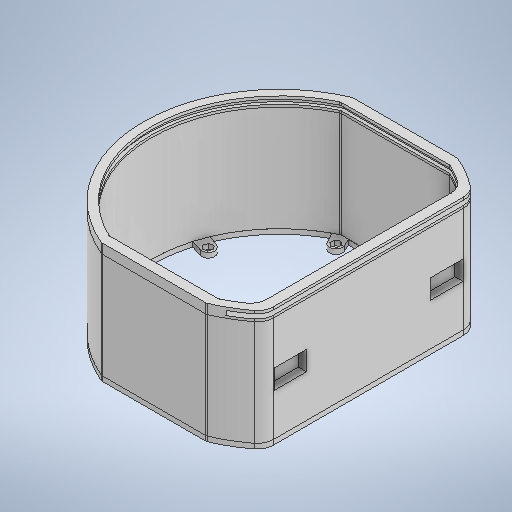
# Autodesk Inventor part: carcasa4.0
Saved by Autodesk Inventor 2025.3 (Build 293356030, 356C)
## iProperties
Created: 2025-08-27
Part Number: carcasa4.0
Material: Generic
Document SubType Name: Modeling
Designer: cdavi
Density: 1 g/cm^3
Appearance: Default
Author: cdavi
Autodesk Inventor part; units mm, degrees
ref_plane "YZ Plane" through (0, 0, 0) normal (1, 0, 0) x (0, 1, 0)
ref_plane "XZ Plane" through (0, 0, 0) normal (0, 1, 0) x (-1, 0, 0)
ref_plane "XY Plane" through (0, 0, 0) normal (0, 0, 1) x (1, 0, 0)
sketch "Sketch1" plane through (0, 0, 0) normal (0, 1, 0) x (-1, 0, 0)
  line L0 (33.1474, 71.5) -> (-33.1474, 71.5)
  line L1 (0, 0) -> (-55, 0) construction
  line L2 (31.9961, 77.5) -> (-31.9961, 77.5)
  line L3 (33.1474, -71.5) -> (-33.5969, -71.5)
  line L4 (31.9961, -77.5) -> (-31.9961, -77.5)
  line L5 (0, 0) -> (0, 77.5) construction
  line L6 (-49, 56.921) -> (-49, -56.921)
  line L7 (-55, 58.7452) -> (-55, -58.7452)
  arc A0 (-44.6522, -65.1704) -> (-33.5969, -71.5) centre (0, 0) ccw
  arc A1 (-51.0811, -66.6838) -> (-32.7765, -77.3415) centre (0, 0) ccw
  arc A2 (32.7765, -77.3415) -> (32.7765, 77.3415) centre (0, 0) ccw
  arc A3 (-32.7765, 77.3415) -> (-51.0811, 66.6838) centre (0, 0) ccw
  arc A4 (34.0084, -71.3052) -> (34.0084, 71.3052) centre (0, 0) ccw
  arc A5 (-34.0084, 71.3052) -> (-44.6522, 65.1704) centre (0, 0) ccw
  arc A6 (-32.7765, -77.3415) -> (-31.9961, -77.5) centre (-31.9961, -75.5) ccw
  arc A7 (31.9961, -77.5) -> (32.7765, -77.3415) centre (31.9961, -75.5) ccw
  arc A8 (33.1474, -71.5) -> (34.0084, -71.3052) centre (33.1474, -69.5) ccw
  arc A9 (34.0084, 71.3052) -> (33.1474, 71.5) centre (33.1474, 69.5) ccw
  arc A10 (32.7765, 77.3415) -> (31.9961, 77.5) centre (31.9961, 75.5) ccw
  arc A11 (-33.1474, 71.5) -> (-34.0084, 71.3052) centre (-33.1474, 69.5) ccw
  arc A12 (-31.9961, 77.5) -> (-32.7765, 77.3415) centre (-31.9961, 75.5) ccw
  arc A13 (-44.6522, 65.1704) -> (-49, 56.921) centre (-39, 56.921) ccw
  arc A14 (-51.0811, 66.6838) -> (-55, 58.7452) centre (-45, 58.7452) ccw
  arc A15 (-55, -58.7452) -> (-51.0811, -66.6838) centre (-45, -58.7452) ccw
  arc A16 (-49, -56.921) -> (-44.6522, -65.1704) centre (-39, -56.921) ccw
  point P0 (-32.3998, 77.5)
  point P1 (33.5969, -71.5)
  point P2 (32.3998, -77.5)
  point P3 (-32.3998, -77.5)
  point P4 (-55, -63.4902)
  point P5 (-49, 61.9677)
  point P6 (-49, -61.9677)
  point P7 (-55, 63.4902)
  point P8 (32.3998, 77.5)
  point P9 (33.5969, 71.5)
  point P10 (-33.5969, 71.5)
  dimension "d2" = 71.5
  dimension "d4" = 6
  dimension "d6" = 49
  dimension "d7" = 6
  dimension "d8" = 2
  dimension "d9" = 10
  dimension "d10" = 79
  dimension "d11" = 84
  dimension "d12" = 79
  dimension "d13" = 84
  constraints: 45 point on circle, 22 tangent, 17 centre point, 16 end point, 11 point on line, 9 equal radius, 4 symmetric about line, 3 vertical, 2 coincident, 2 horizontal, 2 midpoint, 1 parallel
  measures "d2" distance between parallel lines of L1 L0
  measures "d4" distance between parallel lines of L0 L2
  measures "d6" distance between parallel lines of L6 L5
  measures "d7" distance between parallel lines of L7 L6
  measures "d8" radius of A6
  measures "d9" radius of A13
  measures "d10" radius of A4
  measures "d11" radius of A2
  measures "d12" radius of A0
  measures "d13" radius of A1
extrude "Extrusion1" add sketch "Sketch1" along normal blind 65
sketch "Sketch2" plane through (55, 0, 58.7452) normal (1, 0, 0) x (0, 0, -1)
  line L0 (58.7452, 0) -> (58.7452, 65) construction
  line L1 (115.6662, 65) -> (1.8242, 65) projected
  line L2 (0.4037, 38) -> (20.4037, 38)
  line L3 (20.4037, 38) -> (20.4037, 26)
  line L4 (20.4037, 26) -> (0.4037, 26)
  line L5 (0.4037, 26) -> (0.4037, 38)
  line L6 (0, 0) -> (117.4904, 0) projected
  line L7 (-18.5963, 0) -> (-18.5963, 65) projected
  line L8 (117.0867, 38) -> (97.0867, 38)
  line L9 (97.0867, 38) -> (97.0867, 26)
  line L10 (97.0867, 26) -> (117.0867, 26)
  line L11 (117.0867, 26) -> (117.0867, 38)
  dimension "d16" = 26
  dimension "d17" = 19
  dimension "d18" = 12
  dimension "d19" = 20
  constraints: 18 end point, 4 symmetric about line, 2 parallel, 1 horizontal, 1 midpoint, 1 perpendicular
  measures "d16" distance between parallel lines of L6 L4
  measures "d17" distance between parallel lines of L5 L7
  measures "d18" distance of L2.end L3.end
  measures "d19" distance of L2.start L2.end
extrude "Extrusion2" cut sketch "Sketch2" against normal blind 5
sketch "Sketch3" plane through (55, 0, 58.7452) normal (1, 0, 0) x (0, 0, -1)
  line L0 (3.568, 49.2223) -> (17.7975, 43.9952) construction
  line L1 (2.8909, 47.379) -> (17.1204, 42.1519)
  line L2 (18.4746, 45.8385) -> (4.2452, 51.0656)
  arc A0 (4.2452, 51.0656) -> (2.8909, 47.379) centre (3.568, 49.2223) ccw
  arc A1 (17.1204, 42.1519) -> (18.4746, 45.8385) centre (17.7975, 43.9952) ccw
  arc A2 (44.4296, 11.624) -> (34.6921, 2.9774) centre (43.8866, 2.4292) ccw construction
  arc A3 (44.531, 13.3402) -> (32.9759, 3.0797) centre (43.8866, 2.4292) ccw
  arc A4 (44.3283, 9.9077) -> (36.4083, 2.8751) centre (43.8866, 2.4292) ccw
  arc A5 (44.3283, 9.9077) -> (44.531, 13.3402) centre (44.4296, 11.624) ccw
  arc A6 (32.9759, 3.0797) -> (36.4083, 2.8751) centre (34.6921, 2.9774) ccw
  line L3 (58.7452, 0) -> (58.7452, 65) construction
  line L4 (114.5995, 47.379) -> (100.3701, 42.1519)
  line L5 (99.0158, 45.8385) -> (113.2453, 51.0656)
  arc A7 (114.5995, 47.379) -> (113.2453, 51.0656) centre (113.9224, 49.2223) ccw
  arc A8 (99.0158, 45.8385) -> (100.3701, 42.1519) centre (99.6929, 43.9952) ccw
  point P0 (10.6828, 46.6088)
  constraints: 18 point on circle, 12 end point, 9 centre point, 8 tangent, 6 symmetric about line, 1 midpoint, 1 parallel, 2 other
extrude "Extrusion3" [suppressed]
extrude "Extrusion4" add sketch "Sketch1" along normal blind 3 from surface at 65 separate body contours A9 A4 A8 L3 A0 A16 L6 A13 A5 A11 L0 | A10 A2 A7 L4 A6 A1 A15 L7 A14 A3 A12 L2
sketch "Sketch5" plane through (-31.9961, 68, 77.5) normal (0, 1, 0) x (1, 0, 0)
  circle A0 centre (31.9961, 77.5) radius 8.5
  circle A1 centre (1.9961, 77.5) radius 2.5
  line L0 (40.1201, 75) -> (48.9961, 75)
  line L1 (48.9961, 75) -> (48.9961, 80)
  line L2 (48.9961, 80) -> (40.1201, 80)
  line L3 (48.9961, 77.5) -> (86.9961, 77.5)
  line L4 (86.9961, 18.7548) -> (86.9961, 136.2452) projected
  line L5 (1.9961, 77.5) -> (-52.0039, 77.5)
  arc A2 (-0.7804, 154.8415) -> (-0.7804, 0.1585) centre (31.9961, 77.5) ccw projected
  dimension "d26" = 17
  dimension "d27" = 5
  dimension "d31" = 5
  dimension "d32" = 17
  dimension "d47" = 30
  dimension "d204" = 38
  dimension "d205" = 54
  dimension "d206" = 55
  constraints: 10 end point, 3 point on circle, 2 centre point, 2 horizontal alignment, 2 midpoint, 2 perpendicular, 1 coincident, 1 horizontal, 1 point on line
  measures "d26" diameter of A0
  measures "d27" diameter of A1
  measures "d31" distance between parallel lines of L2 L0
  measures "d32" distance from line of A0.centre L1
  measures "d47" distance of A0.centre L5.start
  measures "d204" distance of L3.start L3.end
  measures "d205" distance of L5.start L5.end
  measures "d206" distance from line of L4 point (31.996, 77.5)
extrude "Extrusion5" cut sketch "Sketch5" against normal through all bodies 2
sketch "Sketch6" plane through (0, 0, 0) normal (0, 1, 0) x (-1, 0, 0)
  circle A0 centre (0, 0) radius 72 construction
  arc A1 (-34.0084, 71.3052) -> (-44.6522, 65.1704) centre (0, 0) ccw projected
  arc A2 (-44.6522, 65.1704) -> (-49, 56.921) centre (-39, 56.921) ccw projected
  line L0 (-49, -56.921) -> (-49, 56.921) projected
  arc A3 (-49, -56.921) -> (-44.6522, -65.1704) centre (-39, -56.921) ccw projected
  arc A4 (-44.6522, -65.1704) -> (-33.5969, -71.5) centre (0, 0) ccw projected
  line L1 (33.1474, -71.5) -> (-33.5969, -71.5) construction
  arc A5 (34.0084, -71.3052) -> (34.0084, 71.3052) centre (0, 0) ccw projected
  line L2 (-33.1474, 71.5) -> (33.1474, 71.5) construction
  line L3 (31.9961, 77.5) -> (-31.9961, 77.5) projected
  arc A6 (-32.7765, 77.3415) -> (-51.0811, 66.6838) centre (0, 0) ccw projected
  arc A7 (-51.0811, 66.6838) -> (-55, 58.7452) centre (-45, 58.7452) ccw projected
  line L4 (-55, 58.7452) -> (-55, -58.7452) projected
  arc A8 (-55, -58.7452) -> (-51.0811, -66.6838) centre (-45, -58.7452) ccw projected
  arc A9 (-51.0811, -66.6838) -> (-32.7765, -77.3415) centre (0, 0) ccw projected
  line L5 (-31.9961, -77.5) -> (31.9961, -77.5) projected
  arc A10 (32.7765, -77.3415) -> (32.7765, 77.3415) centre (0, 0) ccw projected
  arc A11 (-32.6555, 65.2887) -> (-41.2609, 60.2208) centre (0, 0) ccw construction
  arc A12 (-41.2609, 60.2208) -> (-43, 56.921) centre (-39, 56.921) ccw construction
  line L6 (-43, 56.921) -> (-43, -56.921) construction
  arc A13 (-43, -56.921) -> (-41.2609, -60.2208) centre (-39, -56.921) ccw construction
  arc A14 (-41.2609, -60.2208) -> (-32.6555, -65.2887) centre (0, 0) ccw construction
  line L7 (-31.7608, -65.5) -> (31.7608, -65.5) construction
  line L8 (-31.7608, 65.5) -> (31.7608, 65.5) construction
  arc A15 (32.6555, -65.2887) -> (32.6555, 65.2887) centre (0, 0) ccw construction
  arc A16 (-8.124, -2.5) -> (-8.124, 2.5) centre (0, 0) ccw projected
  line L9 (0, 0) -> (67.9077, 23.9278) construction
  line L10 (0, 0) -> (84, 0) construction
  circle A17 centre (67.9077, 23.9278) radius 2.85 construction
  line L11 (0, 0) -> (0, -72) construction
  circle A18 centre (30.4285, 65.2542) radius 2.85 construction
  line L12 (30.4285, 65.2542) -> (0, 0) construction
  circle A19 centre (-45.5, 20) radius 2.85 construction
  circle A20 centre (-30.4285, 65.2542) radius 2.85 construction
  line L13 (-30.4285, 65.2542) -> (0, 0) construction
  arc A21 (-31.7608, 65.5) -> (-32.6555, 65.2887) centre (-31.7608, 63.5) ccw construction
  arc A22 (-32.6555, -65.2887) -> (-31.7608, -65.5) centre (-31.7608, -63.5) ccw construction
  arc A23 (31.7608, -65.5) -> (32.6555, -65.2887) centre (31.7608, -63.5) ccw construction
  arc A24 (32.6555, 65.2887) -> (31.7608, 65.5) centre (31.7608, 63.5) ccw construction
  arc A25 (-32.7765, -77.3415) -> (-31.9961, -77.5) centre (-31.9961, -75.5) ccw projected
  arc A26 (31.9961, -77.5) -> (32.7765, -77.3415) centre (31.9961, -75.5) ccw projected
  arc A27 (32.7765, 77.3415) -> (31.9961, 77.5) centre (31.9961, 75.5) ccw projected
  arc A28 (-31.9961, 77.5) -> (-32.7765, 77.3415) centre (-31.9961, 75.5) ccw projected
  circle A29 centre (67.9077, -23.9278) radius 2.85 construction
  circle A30 centre (30.4285, -65.2542) radius 2.85 construction
  circle A31 centre (-45.5, -20) radius 2.85 construction
  circle A32 centre (-30.4285, -65.2542) radius 2.85 construction
  line L14 (34.0084, 64.5944) -> (34.0084, 71.3052)
  line L15 (-34.0084, 64.5944) -> (-34.0084, 71.3052)
  line L16 (34.0084, 71.3052) -> (-34.0084, 71.3052)
  line L17 (34.0084, -64.5944) -> (34.0084, -71.3052)
  line L18 (-34.0084, -64.5944) -> (-34.0084, -71.3052)
  line L19 (34.0084, -71.3052) -> (-34.0084, -71.3052)
  circle A33 centre (67.9077, 23.9278) radius 4
  circle A34 centre (30.4285, 65.2542) radius 4
  line L20 (65.1063, 24.4516) -> (66.9606, 26.6158)
  line L21 (66.9606, 26.6158) -> (69.762, 26.0921)
  line L22 (69.762, 26.0921) -> (70.7092, 23.4041)
  line L23 (70.7092, 23.4041) -> (68.8549, 21.2398)
  line L24 (68.8549, 21.2398) -> (66.0534, 21.7636)
  line L25 (66.0534, 21.7636) -> (65.1063, 24.4516)
  line L26 (28.0939, 63.6195) -> (27.8455, 66.4586)
  line L27 (27.8455, 66.4586) -> (30.1801, 68.0933)
  line L28 (30.1801, 68.0933) -> (32.7631, 66.8889)
  line L29 (32.7631, 66.8889) -> (33.0115, 64.0497)
  line L30 (33.0115, 64.0497) -> (30.6769, 62.415)
  line L31 (30.6769, 62.415) -> (28.0939, 63.6195)
  circle A35 centre (-45.5, 20) radius 4
  line L32 (-47.9682, 18.575) -> (-47.9682, 21.425)
  line L33 (-47.9682, 21.425) -> (-45.5, 22.85)
  line L34 (-45.5, 22.85) -> (-43.0318, 21.425)
  line L35 (-43.0318, 21.425) -> (-43.0318, 18.575)
  line L36 (-43.0318, 18.575) -> (-45.5, 17.15)
  line L37 (-45.5, 17.15) -> (-47.9682, 18.575)
  line L38 (-45.5, 24) -> (-49, 24)
  line L39 (-45.5, 16) -> (-49, 16)
  circle A36 centre (-30.4285, 65.2542) radius 4
  line L40 (-30.6769, 62.415) -> (-33.0115, 64.0497)
  line L41 (-33.0115, 64.0497) -> (-32.7631, 66.8889)
  line L42 (-32.7631, 66.8889) -> (-30.1801, 68.0933)
  line L43 (-30.1801, 68.0933) -> (-27.8455, 66.4586)
  line L44 (-27.8455, 66.4586) -> (-28.0939, 63.6195)
  line L45 (-28.0939, 63.6195) -> (-30.6769, 62.415)
  line L46 (-34.0054, 63.4636) -> (-37.1399, 69.7254)
  circle A37 centre (67.9077, -23.9278) radius 4
  circle A38 centre (30.4285, -65.2542) radius 4
  circle A39 centre (-45.5, -20) radius 4
  line L47 (-45.5, -24) -> (-49, -24)
  line L48 (-45.5, -16) -> (-49, -16)
  circle A40 centre (-30.4285, -65.2542) radius 4
  line L49 (-34.0054, -63.4636) -> (-37.1399, -69.7254)
  line L50 (65.1063, -24.4516) -> (66.9606, -26.6158)
  line L51 (66.9606, -26.6158) -> (69.762, -26.0921)
  line L52 (69.762, -26.0921) -> (70.7092, -23.4041)
  line L53 (70.7092, -23.4041) -> (68.8549, -21.2398)
  line L54 (68.8549, -21.2398) -> (66.0534, -21.7636)
  line L55 (66.0534, -21.7636) -> (65.1063, -24.4516)
  line L56 (28.0939, -63.6195) -> (27.8455, -66.4586)
  line L57 (27.8455, -66.4586) -> (30.1801, -68.0933)
  line L58 (30.1801, -68.0933) -> (32.7631, -66.8889)
  line L59 (32.7631, -66.8889) -> (33.0115, -64.0497)
  line L60 (33.0115, -64.0497) -> (30.6769, -62.415)
  line L61 (30.6769, -62.415) -> (28.0939, -63.6195)
  line L62 (-30.6769, -62.415) -> (-33.0115, -64.0497)
  line L63 (-33.0115, -64.0497) -> (-32.7631, -66.8889)
  line L64 (-32.7631, -66.8889) -> (-30.1801, -68.0933)
  line L65 (-30.1801, -68.0933) -> (-27.8455, -66.4586)
  line L66 (-27.8455, -66.4586) -> (-28.0939, -63.6195)
  line L67 (-28.0939, -63.6195) -> (-30.6769, -62.415)
  line L68 (-47.9682, -18.575) -> (-47.9682, -21.425)
  line L69 (-47.9682, -21.425) -> (-45.5, -22.85)
  line L70 (-45.5, -22.85) -> (-43.0318, -21.425)
  line L71 (-43.0318, -21.425) -> (-43.0318, -18.575)
  line L72 (-43.0318, -18.575) -> (-45.5, -17.15)
  line L73 (-45.5, -17.15) -> (-47.9682, -18.575)
  line L74 (66.4741, 27.6621) -> (73.0114, 30.1718)
  line L75 (69.1317, 20.1197) -> (75.7983, 22.2625)
  line L76 (34.0054, 63.4636) -> (37.1399, 69.7254)
  line L77 (66.4741, -27.6621) -> (73.0114, -30.1718)
  line L78 (69.1317, -20.1197) -> (75.7983, -22.2625)
  line L79 (34.0054, -63.4636) -> (37.1399, -69.7254)
  line L80 (-26.7577, 66.8433) -> (-29.5397, 73.2694)
  line L81 (26.7577, 66.8433) -> (29.5397, 73.2694)
  line L82 (-26.7577, -66.8433) -> (-29.5397, -73.2694)
  line L83 (26.7577, -66.8433) -> (29.5397, -73.2694)
  line L84 (-33.1474, 71.5) -> (-55, 71.5)
  line L85 (-55, 71.5) -> (-55, 58.7452)
  line L86 (-44.088, 71.5) -> (-33.1474, 71.5)
  point P0 (-32.2296, -65.5)
  point P1 (-34.0084, 64.5944)
  point P2 (30.4285, 65.2542)
  point P3 (-37.1399, -69.7254)
  point P4 (-49, -24)
  point P5 (-49, -16)
  point P6 (75.7983, -22.2625)
  point P7 (69.1317, -20.1197)
  point P8 (66.4741, -27.6621)
  point P9 (73.0114, -30.1718)
  point P10 (34.0054, -63.4636)
  point P11 (-27.1107, 64.5369)
  point P12 (-27.1107, -64.5369)
  point P13 (27.1107, -64.5369)
  point P14 (27.1107, 64.5369)
  point P15 (-49, 21.9365)
  point P16 (-49, 18.0635)
  point P17 (-32.0117, 62.2515)
  point P18 (32.0117, -62.2515)
  point P19 (66.8707, -20.6956)
  point P20 (65.0736, -25.796)
  point P21 (-32.0117, -62.2515)
  point P22 (-49, -21.9365)
  point P23 (-49, -18.0635)
  point P24 (65.0736, 25.796)
  point P25 (66.8707, 20.6956)
  point P26 (32.0117, 62.2515)
  point P27 (25.828, -65.0609)
  point P28 (-25.828, -65.0609)
  point P29 (-26.7577, -66.8433)
  point P30 (34.0084, -67.0387)
  point P31 (-28.6893, -71.3052)
  point P32 (28.6893, -71.3052)
  point P33 (28.6893, 71.3052)
  point P34 (-28.6893, 71.3052)
  point P35 (34.0084, 67.0387)
  point P36 (-34.0084, -71.3052)
  point P37 (-34.0084, -67.0387)
  point P38 (-34.0084, 67.0387)
  dimension "d33" = 144
  dimension "d39" = 5.7
  dimension "d34" = 6
  dimension "d35" = 6
  dimension "d36" = 6
  dimension "d37" = 19.41
  dimension "d38" = 25
  dimension "d40" = 20
  dimension "d41" = 3.5
  dimension "d42" = 25
  dimension "d44" = 2
  dimension "d61" = 8
  dimension "d62" = 8
  dimension "d63" = 8
  dimension "d64" = 8
  dimension "d171" = 90
  dimension "d172" = 12.7548
  constraints: 162 end point, 52 symmetric about line, 38 point on circle, 20 centre point, 16 tangent, 10 coincident, 6 perpendicular, 4 point on line, 3 equal radius, 2 parallel, 2 vertical, 1 collinear, 1 horizontal, 93 other
  measures "d34" radial gap between concentric circles of A1 A11
  measures "d35" distance between parallel lines of L2 L8
  measures "d36" radial gap between concentric circles of A5 A15
  measures "d37" angle of L10 L9
  measures "d38" angle of L11 L12
  measures "d40" distance from line of point (-45.5, 20) L10
  measures "d41" distance from line of L0 point (-45.5, 20)
  measures "d42" angle of L11 L13
  measures "d44" radius of A21
  measures "d61" diameter of A33
  measures "d62" diameter of A34
  measures "d63" diameter of A35
  measures "d64" diameter of A36
  measures "d171" angle of L85 L84
  measures "d172" distance of L84.end L4.start
extrude "Extrusion6" add sketch "Sketch6" against normal blind 3 separate body contours L15 A36 L46 A1 | L16 L80 A36 L15 | A36 | L16 L14 A34 L81 | A5 L76 A34 L14 | A34 | L38 A35 L0 | A35 L0 | L0 A35 | A5 L75 A33 L74 | A35 L39 L0 | A33 | A5 L77 A37 L78 | L48 A39 L0 | A37 | A39 L0 | L0 A39 | A5 L17 A38 L79 | A39 L47 L0 | L19 L83 A38 L17 | A38 | L19 L18 A40 L82 | A4 L49 A40 L18 | A40 | A27 A10 A26 L5 A25 A9 A8 L4 A7 A6 A28 L3
sketch "Sketch14" plane through (0, 65, 0) normal (0, 1, 0) x (1, 0, 0)
  arc A0 (-32.7765, 77.3415) -> (-32.7765, -77.3415) centre (0, 0) ccw projected
  arc A1 (-32.7765, -77.3415) -> (-31.9961, -77.5) centre (-31.9961, -75.5) ccw projected
  line L0 (-31.9961, -77.5) -> (31.9961, -77.5) projected
  arc A2 (31.9961, -77.5) -> (32.7765, -77.3415) centre (31.9961, -75.5) ccw projected
  arc A3 (32.7765, -77.3415) -> (51.0811, -66.6838) centre (0, 0) ccw projected
  arc A4 (51.0811, -66.6838) -> (55, -58.7452) centre (45, -58.7452) ccw projected
  line L1 (55, -58.7452) -> (55, 58.7452) projected
  arc A5 (55, 58.7452) -> (51.0811, 66.6838) centre (45, 58.7452) ccw projected
  arc A6 (51.0811, 66.6838) -> (32.7765, 77.3415) centre (0, 0) ccw projected
  arc A7 (32.7765, 77.3415) -> (31.9961, 77.5) centre (31.9961, 75.5) ccw projected
  line L2 (31.9961, 77.5) -> (-31.9961, 77.5) projected
  arc A8 (-31.9961, 77.5) -> (-32.7765, 77.3415) centre (-31.9961, 75.5) ccw projected
  line L3 (-33.1474, 71.5) -> (33.5969, 71.5) projected
  arc A9 (44.6522, 65.1704) -> (33.5969, 71.5) centre (0, 0) ccw projected
  arc A10 (49, 56.921) -> (44.6522, 65.1704) centre (39, 56.921) ccw projected
  line L4 (49, 56.921) -> (49, -56.921) projected
  arc A11 (44.6522, -65.1704) -> (49, -56.921) centre (39, -56.921) ccw projected
  arc A12 (34.0084, -71.3052) -> (44.6522, -65.1704) centre (0, 0) ccw projected
  arc A13 (33.1474, -71.5) -> (34.0084, -71.3052) centre (33.1474, -69.5) ccw projected
  line L5 (33.1474, -71.5) -> (-33.1474, -71.5) projected
  arc A14 (-34.0084, -71.3052) -> (-33.1474, -71.5) centre (-33.1474, -69.5) ccw projected
  arc A15 (-34.0084, 71.3052) -> (-34.0084, -71.3052) centre (0, 0) ccw projected
  arc A16 (-33.1474, 71.5) -> (-34.0084, 71.3052) centre (-33.1474, 69.5) ccw projected
extrude "Extrusion11" add sketch "Sketch14" along normal blind 6 separate body
sketch "Sketch15" plane through (55, 65, 58.7452) normal (1, 0, 0) x (0, 0, -1)
  line L0 (58.7452, 6) -> (58.7452, 0)
  line L1 (58.7452, 6) -> (0, 6)
  line L2 (0, 6) -> (-14.763, 6)
  line L3 (-14.763, 6) -> (-14.763, 0)
  line L4 (-14.763, 0) -> (0, 0)
  line L5 (0, 0) -> (58.7452, 0)
  line L6 (1.8242, 0) -> (58.7452, 0)
  line L7 (58.7452, 6) -> (0, 6)
  line L8 (58.7452, 6) -> (58.7452, 4.5)
  line L9 (58.7452, 4.5) -> (0, 4.246)
  line L10 (0, 0) -> (0, 6) projected
  line L11 (58.7452, 0) -> (58.7452, 1.5)
  line L12 (58.7452, 1.5) -> (0, 1.5)
  arc A0 (58.7452, 4.5) -> (58.7452, 4.5) centre (58.0571, 163.658) ccw
  line L13 (0, 4.246) -> (-14.763, 4.246)
  line L14 (0, 1.5) -> (-14.763, 1.5)
  line L15 (58.7452, 6) -> (117.4904, 6)
  line L16 (117.4904, 6) -> (132.2534, 6)
  line L17 (132.2534, 6) -> (132.2534, 0)
  line L18 (132.2534, 0) -> (117.4904, 0)
  line L19 (117.4904, 0) -> (58.7452, 0)
  line L20 (115.6662, 0) -> (58.7452, 0)
  line L21 (58.7452, 6) -> (117.4904, 6)
  line L22 (58.7452, 4.5) -> (117.4904, 4.246)
  line L23 (117.4904, 0) -> (117.4904, 6)
  line L24 (58.7452, 1.5) -> (117.4904, 1.5)
  arc A1 (58.7452, 4.5) -> (58.7452, 4.5) centre (59.4334, 163.658) ccw
  line L25 (117.4904, 4.246) -> (132.2534, 4.246)
  line L26 (117.4904, 1.5) -> (132.2534, 1.5)
  point P0 (58.7452, -65)
  dimension "d173" = 14.763
  dimension "d176" = 1.5
  dimension "d177" = 1.5
  dimension "d202" = 2.746
  constraints: 52 end point, 15 point on line, 11 symmetric about line, 6 perpendicular, 4 point on circle, 2 centre point, 1 collinear, 1 tangent, 1 other
  measures "d173" distance of L1.end L2.end
  measures "d176" distance of L0.start L8.end
  measures "d177" distance of L0.end L11.end
  measures "d202" distance between parallel lines of L14 L13
extrude "Extrusion12" cut sketch "Sketch15" against normal blind 89.021 contours L22 L23 L24 L0 | L0 L12 L10 L9 | L10 L14 L3 L13 | L25 L17 L26 L23 bodies 4
ref_plane "Work Plane1" through (0, 66.5, 0) normal (0, -1, 0) x (1, 0, 0)
sketch "Sketch18" plane through (0, 66.5, 0) normal (0, -1, 0) x (1, 0, 0)
  arc A0 (33.5969, -71.5) -> (44.6522, -65.1704) centre (0, 0) ccw projected
  arc A1 (-34.021, 71.2992) -> (-34.021, -71.2992) centre (0, 0) ccw
  arc A2 (-34.021, 73.509) -> (-34.021, -73.509) centre (0, 0) ccw
  line L0 (-34.021, 71.2992) -> (-34.021, 73.509)
  line L1 (-34.021, -71.2992) -> (-34.021, -73.509)
  point P0 (-34.0084, 71.3052)
  point P1 (-34.021, -73.5082)
  dimension "d209" = 162
  constraints: 5 point on circle, 4 end point, 2 centre point, 2 vertical, 1 coincident
  measures "d209" diameter of A2
extrude "Extrusion14" cut sketch "Sketch18" against normal blind 2.746 bodies 4
body "Solid1"
body "Solid2"
body "Solid3"
body "Solid4"
